Autodesk Inventor part; units mm, degrees
(part 2 of 4)
sketch "Sketch18" plane through (0, 4, 0) normal (0, 1, 0) x (1, 0, 0)
  line L0 (-39.75, -116.5) -> (-38.25, -116.5)
  line L1 (-38.25, -116.5) -> (-38.25, -108.5)
  line L2 (-38.25, -108.5) -> (-39.75, -108.5)
  line L3 (-39.75, -108.5) -> (-39.75, -116.5)
  line L4 (-41, -119.5) -> (-49.5, -119.5) projected
  line L5 (-41, -118) -> (-41, -119.5) projected
  line L6 (-24.75, -116.5) -> (-23.25, -116.5)
  line L7 (-23.25, -116.5) -> (-23.25, -108.5)
  line L8 (-23.25, -108.5) -> (-24.75, -108.5)
  line L9 (-24.75, -108.5) -> (-24.75, -116.5)
  line L10 (-9.75, -116.5) -> (-8.25, -116.5)
  line L11 (-8.25, -116.5) -> (-8.25, -108.5)
  line L12 (-8.25, -108.5) -> (-9.75, -108.5)
  line L13 (-9.75, -108.5) -> (-9.75, -116.5)
  line L14 (5.25, -116.5) -> (6.75, -116.5)
  line L15 (6.75, -116.5) -> (6.75, -108.5)
  line L16 (6.75, -108.5) -> (5.25, -108.5)
  line L17 (5.25, -108.5) -> (5.25, -116.5)
  line L18 (20.25, -116.5) -> (21.75, -116.5)
  line L19 (21.75, -116.5) -> (21.75, -108.5)
  line L20 (21.75, -108.5) -> (20.25, -108.5)
  line L21 (20.25, -108.5) -> (20.25, -116.5)
  line L22 (35.25, -116.5) -> (36.75, -116.5)
  line L23 (36.75, -116.5) -> (36.75, -108.5)
  line L24 (36.75, -108.5) -> (35.25, -108.5)
  line L25 (35.25, -108.5) -> (35.25, -116.5)
  line L26 (50.25, -116.5) -> (51.75, -116.5)
  line L27 (51.75, -116.5) -> (51.75, -108.5)
  line L28 (51.75, -108.5) -> (50.25, -108.5)
  line L29 (50.25, -108.5) -> (50.25, -116.5)
  line L30 (-39.75, -101.5) -> (-38.25, -101.5)
  line L31 (-38.25, -101.5) -> (-38.25, -93.5)
  line L32 (-38.25, -93.5) -> (-39.75, -93.5)
  line L33 (-39.75, -93.5) -> (-39.75, -101.5)
  line L34 (-24.75, -101.5) -> (-23.25, -101.5)
  line L35 (-23.25, -101.5) -> (-23.25, -93.5)
  line L36 (-23.25, -93.5) -> (-24.75, -93.5)
  line L37 (-24.75, -93.5) -> (-24.75, -101.5)
  line L38 (-9.75, -101.5) -> (-8.25, -101.5)
  line L39 (-8.25, -101.5) -> (-8.25, -93.5)
  line L40 (-8.25, -93.5) -> (-9.75, -93.5)
  line L41 (-9.75, -93.5) -> (-9.75, -101.5)
  line L42 (5.25, -101.5) -> (6.75, -101.5)
  line L43 (6.75, -101.5) -> (6.75, -93.5)
  line L44 (6.75, -93.5) -> (5.25, -93.5)
  line L45 (5.25, -93.5) -> (5.25, -101.5)
  line L46 (20.25, -101.5) -> (21.75, -101.5)
  line L47 (21.75, -101.5) -> (21.75, -93.5)
  line L48 (21.75, -93.5) -> (20.25, -93.5)
  line L49 (20.25, -93.5) -> (20.25, -101.5)
  line L50 (35.25, -101.5) -> (36.75, -101.5)
  line L51 (36.75, -101.5) -> (36.75, -93.5)
  line L52 (36.75, -93.5) -> (35.25, -93.5)
  line L53 (35.25, -93.5) -> (35.25, -101.5)
  line L54 (50.25, -101.5) -> (51.75, -101.5)
  line L55 (51.75, -101.5) -> (51.75, -93.5)
  line L56 (51.75, -93.5) -> (50.25, -93.5)
  line L57 (50.25, -93.5) -> (50.25, -101.5)
  line L58 (-39.75, -86.5) -> (-38.25, -86.5)
  line L59 (-38.25, -86.5) -> (-38.25, -78.5)
  line L60 (-38.25, -78.5) -> (-39.75, -78.5)
  line L61 (-39.75, -78.5) -> (-39.75, -86.5)
  line L62 (-24.75, -86.5) -> (-23.25, -86.5)
  line L63 (-23.25, -86.5) -> (-23.25, -78.5)
  line L64 (-23.25, -78.5) -> (-24.75, -78.5)
  line L65 (-24.75, -78.5) -> (-24.75, -86.5)
  line L66 (-9.75, -86.5) -> (-8.25, -86.5)
  line L67 (-8.25, -86.5) -> (-8.25, -78.5)
  line L68 (-8.25, -78.5) -> (-9.75, -78.5)
  line L69 (-9.75, -78.5) -> (-9.75, -86.5)
  line L70 (5.25, -86.5) -> (6.75, -86.5)
  line L71 (6.75, -86.5) -> (6.75, -78.5)
  line L72 (6.75, -78.5) -> (5.25, -78.5)
  line L73 (5.25, -78.5) -> (5.25, -86.5)
  line L74 (20.25, -86.5) -> (21.75, -86.5)
  line L75 (21.75, -86.5) -> (21.75, -78.5)
  line L76 (21.75, -78.5) -> (20.25, -78.5)
  line L77 (20.25, -78.5) -> (20.25, -86.5)
  line L78 (35.25, -86.5) -> (36.75, -86.5)
  line L79 (36.75, -86.5) -> (36.75, -78.5)
  line L80 (36.75, -78.5) -> (35.25, -78.5)
  line L81 (35.25, -78.5) -> (35.25, -86.5)
  line L82 (50.25, -86.5) -> (51.75, -86.5)
  line L83 (51.75, -86.5) -> (51.75, -78.5)
  line L84 (51.75, -78.5) -> (50.25, -78.5)
  line L85 (50.25, -78.5) -> (50.25, -86.5)
  line L86 (-39.75, -71.5) -> (-38.25, -71.5)
  line L87 (-38.25, -71.5) -> (-38.25, -63.5)
  line L88 (-38.25, -63.5) -> (-39.75, -63.5)
  line L89 (-39.75, -63.5) -> (-39.75, -71.5)
  line L90 (-24.75, -71.5) -> (-23.25, -71.5)
  line L91 (-23.25, -71.5) -> (-23.25, -63.5)
  line L92 (-23.25, -63.5) -> (-24.75, -63.5)
  line L93 (-24.75, -63.5) -> (-24.75, -71.5)
  line L94 (-9.75, -71.5) -> (-8.25, -71.5)
  line L95 (-8.25, -71.5) -> (-8.25, -63.5)
  line L96 (-8.25, -63.5) -> (-9.75, -63.5)
  line L97 (-9.75, -63.5) -> (-9.75, -71.5)
  line L98 (5.25, -71.5) -> (6.75, -71.5)
  line L99 (6.75, -71.5) -> (6.75, -63.5)
  line L100 (6.75, -63.5) -> (5.25, -63.5)
  line L101 (5.25, -63.5) -> (5.25, -71.5)
  line L102 (20.25, -71.5) -> (21.75, -71.5)
  line L103 (21.75, -71.5) -> (21.75, -63.5)
  line L104 (21.75, -63.5) -> (20.25, -63.5)
  line L105 (20.25, -63.5) -> (20.25, -71.5)
  line L106 (35.25, -71.5) -> (36.75, -71.5)
  line L107 (36.75, -71.5) -> (36.75, -63.5)
  line L108 (36.75, -63.5) -> (35.25, -63.5)
  line L109 (35.25, -63.5) -> (35.25, -71.5)
  line L110 (50.25, -71.5) -> (51.75, -71.5)
  line L111 (51.75, -71.5) -> (51.75, -63.5)
  line L112 (51.75, -63.5) -> (50.25, -63.5)
  line L113 (50.25, -63.5) -> (50.25, -71.5)
  line L114 (-39.75, -56.5) -> (-38.25, -56.5)
  line L115 (-38.25, -56.5) -> (-38.25, -48.5)
  line L116 (-38.25, -48.5) -> (-39.75, -48.5)
  line L117 (-39.75, -48.5) -> (-39.75, -56.5)
  line L118 (-24.75, -56.5) -> (-23.25, -56.5)
  line L119 (-23.25, -56.5) -> (-23.25, -48.5)
  line L120 (-23.25, -48.5) -> (-24.75, -48.5)
  line L121 (-24.75, -48.5) -> (-24.75, -56.5)
  line L122 (-9.75, -56.5) -> (-8.25, -56.5)
  line L123 (-8.25, -56.5) -> (-8.25, -48.5)
  line L124 (-8.25, -48.5) -> (-9.75, -48.5)
  line L125 (-9.75, -48.5) -> (-9.75, -56.5)
  line L126 (5.25, -56.5) -> (6.75, -56.5)
  line L127 (6.75, -56.5) -> (6.75, -48.5)
  line L128 (6.75, -48.5) -> (5.25, -48.5)
  line L129 (5.25, -48.5) -> (5.25, -56.5)
  line L130 (20.25, -56.5) -> (21.75, -56.5)
  line L131 (21.75, -56.5) -> (21.75, -48.5)
  line L132 (21.75, -48.5) -> (20.25, -48.5)
  line L133 (20.25, -48.5) -> (20.25, -56.5)
  line L134 (35.25, -56.5) -> (36.75, -56.5)
  line L135 (36.75, -56.5) -> (36.75, -48.5)
  line L136 (36.75, -48.5) -> (35.25, -48.5)
  line L137 (35.25, -48.5) -> (35.25, -56.5)
  line L138 (50.25, -56.5) -> (51.75, -56.5)
  line L139 (51.75, -56.5) -> (51.75, -48.5)
  line L140 (51.75, -48.5) -> (50.25, -48.5)
  line L141 (50.25, -48.5) -> (50.25, -56.5)
  line L142 (-39.75, -41.5) -> (-38.25, -41.5)
  line L143 (-38.25, -41.5) -> (-38.25, -33.5)
  line L144 (-38.25, -33.5) -> (-39.75, -33.5)
  line L145 (-39.75, -33.5) -> (-39.75, -41.5)
  line L146 (-24.75, -41.5) -> (-23.25, -41.5)
  line L147 (-23.25, -41.5) -> (-23.25, -33.5)
  line L148 (-23.25, -33.5) -> (-24.75, -33.5)
  line L149 (-24.75, -33.5) -> (-24.75, -41.5)
  line L150 (-9.75, -41.5) -> (-8.25, -41.5)
  line L151 (-8.25, -41.5) -> (-8.25, -33.5)
  line L152 (-8.25, -33.5) -> (-9.75, -33.5)
  line L153 (-9.75, -33.5) -> (-9.75, -41.5)
  line L154 (5.25, -41.5) -> (6.75, -41.5)
  line L155 (6.75, -41.5) -> (6.75, -33.5)
  line L156 (6.75, -33.5) -> (5.25, -33.5)
  line L157 (5.25, -33.5) -> (5.25, -41.5)
  line L158 (20.25, -41.5) -> (21.75, -41.5)
  line L159 (21.75, -41.5) -> (21.75, -33.5)
  line L160 (21.75, -33.5) -> (20.25, -33.5)
  line L161 (20.25, -33.5) -> (20.25, -41.5)
  line L162 (35.25, -41.5) -> (36.75, -41.5)
  line L163 (36.75, -41.5) -> (36.75, -33.5)
  line L164 (36.75, -33.5) -> (35.25, -33.5)
  line L165 (35.25, -33.5) -> (35.25, -41.5)
  line L166 (50.25, -41.5) -> (51.75, -41.5)
  line L167 (51.75, -41.5) -> (51.75, -33.5)
  line L168 (51.75, -33.5) -> (50.25, -33.5)
  line L169 (50.25, -33.5) -> (50.25, -41.5)
  line L170 (-39.75, -26.5) -> (-38.25, -26.5)
  line L171 (-38.25, -26.5) -> (-38.25, -18.5)
  line L172 (-38.25, -18.5) -> (-39.75, -18.5)
  line L173 (-39.75, -18.5) -> (-39.75, -26.5)
  line L174 (-24.75, -26.5) -> (-23.25, -26.5)
  line L175 (-23.25, -26.5) -> (-23.25, -18.5)
  line L176 (-23.25, -18.5) -> (-24.75, -18.5)
  line L177 (-24.75, -18.5) -> (-24.75, -26.5)
  line L178 (-9.75, -26.5) -> (-8.25, -26.5)
  line L179 (-8.25, -26.5) -> (-8.25, -18.5)
  line L180 (-8.25, -18.5) -> (-9.75, -18.5)
  line L181 (-9.75, -18.5) -> (-9.75, -26.5)
  line L182 (5.25, -26.5) -> (6.75, -26.5)
  line L183 (6.75, -26.5) -> (6.75, -18.5)
  line L184 (6.75, -18.5) -> (5.25, -18.5)
  line L185 (5.25, -18.5) -> (5.25, -26.5)
  line L186 (20.25, -26.5) -> (21.75, -26.5)
  line L187 (21.75, -26.5) -> (21.75, -18.5)
  line L188 (21.75, -18.5) -> (20.25, -18.5)
  line L189 (20.25, -18.5) -> (20.25, -26.5)
  line L190 (35.25, -26.5) -> (36.75, -26.5)
  line L191 (36.75, -26.5) -> (36.75, -18.5)
  line L192 (36.75, -18.5) -> (35.25, -18.5)
  line L193 (35.25, -18.5) -> (35.25, -26.5)
  line L194 (50.25, -26.5) -> (51.75, -26.5)
  line L195 (51.75, -26.5) -> (51.75, -18.5)
  line L196 (51.75, -18.5) -> (50.25, -18.5)
  line L197 (50.25, -18.5) -> (50.25, -26.5)
  line L198 (-39.75, -11.5) -> (-38.25, -11.5)
  line L199 (-38.25, -11.5) -> (-38.25, -3.5)
  line L200 (-38.25, -3.5) -> (-39.75, -3.5)
  line L201 (-39.75, -3.5) -> (-39.75, -11.5)
  line L202 (-24.75, -11.5) -> (-23.25, -11.5)
  line L203 (-23.25, -11.5) -> (-23.25, -3.5)
  line L204 (-23.25, -3.5) -> (-24.75, -3.5)
  line L205 (-24.75, -3.5) -> (-24.75, -11.5)
  line L206 (-9.75, -11.5) -> (-8.25, -11.5)
  line L207 (-8.25, -11.5) -> (-8.25, -3.5)
  line L208 (-8.25, -3.5) -> (-9.75, -3.5)
  line L209 (-9.75, -3.5) -> (-9.75, -11.5)
  line L210 (5.25, -11.5) -> (6.75, -11.5)
  line L211 (6.75, -11.5) -> (6.75, -3.5)
  line L212 (6.75, -3.5) -> (5.25, -3.5)
  line L213 (5.25, -3.5) -> (5.25, -11.5)
  line L214 (20.25, -11.5) -> (21.75, -11.5)
  line L215 (21.75, -11.5) -> (21.75, -3.5)
  line L216 (21.75, -3.5) -> (20.25, -3.5)
  line L217 (20.25, -3.5) -> (20.25, -11.5)
  line L218 (35.25, -11.5) -> (36.75, -11.5)
  line L219 (36.75, -11.5) -> (36.75, -3.5)
  line L220 (36.75, -3.5) -> (35.25, -3.5)
  line L221 (35.25, -3.5) -> (35.25, -11.5)
  line L222 (50.25, -11.5) -> (51.75, -11.5)
  line L223 (51.75, -11.5) -> (51.75, -3.5)
  line L224 (51.75, -3.5) -> (50.25, -3.5)
  line L225 (50.25, -3.5) -> (50.25, -11.5)
  line L226 (-39.75, 3.5) -> (-38.25, 3.5)
  line L227 (-38.25, 3.5) -> (-38.25, 11.5)
  line L228 (-38.25, 11.5) -> (-39.75, 11.5)
  line L229 (-39.75, 11.5) -> (-39.75, 3.5)
  line L230 (-24.75, 3.5) -> (-23.25, 3.5)
  line L231 (-23.25, 3.5) -> (-23.25, 11.5)
  line L232 (-23.25, 11.5) -> (-24.75, 11.5)
  line L233 (-24.75, 11.5) -> (-24.75, 3.5)
  line L234 (-9.75, 3.5) -> (-8.25, 3.5)
  line L235 (-8.25, 3.5) -> (-8.25, 11.5)
  line L236 (-8.25, 11.5) -> (-9.75, 11.5)
  line L237 (-9.75, 11.5) -> (-9.75, 3.5)
  line L238 (5.25, 3.5) -> (6.75, 3.5)
  line L239 (6.75, 3.5) -> (6.75, 11.5)
  line L240 (6.75, 11.5) -> (5.25, 11.5)
  line L241 (5.25, 11.5) -> (5.25, 3.5)
  line L242 (20.25, 3.5) -> (21.75, 3.5)
  line L243 (21.75, 3.5) -> (21.75, 11.5)
  line L244 (21.75, 11.5) -> (20.25, 11.5)
  line L245 (20.25, 11.5) -> (20.25, 3.5)
  line L246 (35.25, 3.5) -> (36.75, 3.5)
  line L247 (36.75, 3.5) -> (36.75, 11.5)
  line L248 (36.75, 11.5) -> (35.25, 11.5)
  line L249 (35.25, 11.5) -> (35.25, 3.5)
  line L250 (50.25, 3.5) -> (51.75, 3.5)
  line L251 (51.75, 3.5) -> (51.75, 11.5)
  line L252 (51.75, 11.5) -> (50.25, 11.5)
  line L253 (50.25, 11.5) -> (50.25, 3.5)
  line L254 (-39.75, 18.5) -> (-38.25, 18.5)
  line L255 (-38.25, 18.5) -> (-38.25, 26.5)
  line L256 (-38.25, 26.5) -> (-39.75, 26.5)
  line L257 (-39.75, 26.5) -> (-39.75, 18.5)
  line L258 (-24.75, 18.5) -> (-23.25, 18.5)
  line L259 (-23.25, 18.5) -> (-23.25, 26.5)
  line L260 (-23.25, 26.5) -> (-24.75, 26.5)
  line L261 (-24.75, 26.5) -> (-24.75, 18.5)
  line L262 (-9.75, 18.5) -> (-8.25, 18.5)
  line L263 (-8.25, 18.5) -> (-8.25, 26.5)
  line L264 (-8.25, 26.5) -> (-9.75, 26.5)
  line L265 (-9.75, 26.5) -> (-9.75, 18.5)
  line L266 (5.25, 18.5) -> (6.75, 18.5)
  line L267 (6.75, 18.5) -> (6.75, 26.5)
  line L268 (6.75, 26.5) -> (5.25, 26.5)
  line L269 (5.25, 26.5) -> (5.25, 18.5)
  line L270 (20.25, 18.5) -> (21.75, 18.5)
  line L271 (21.75, 18.5) -> (21.75, 26.5)
  line L272 (21.75, 26.5) -> (20.25, 26.5)
  line L273 (20.25, 26.5) -> (20.25, 18.5)
  line L274 (35.25, 18.5) -> (36.75, 18.5)
  line L275 (36.75, 18.5) -> (36.75, 26.5)
  line L276 (36.75, 26.5) -> (35.25, 26.5)
  line L277 (35.25, 26.5) -> (35.25, 18.5)
  line L278 (50.25, 18.5) -> (51.75, 18.5)
  line L279 (51.75, 18.5) -> (51.75, 26.5)
  line L280 (51.75, 26.5) -> (50.25, 26.5)
  line L281 (50.25, 26.5) -> (50.25, 18.5)
  line L282 (-39.75, 33.5) -> (-38.25, 33.5)
  line L283 (-38.25, 33.5) -> (-38.25, 41.5)
  line L284 (-38.25, 41.5) -> (-39.75, 41.5)
  line L285 (-39.75, 41.5) -> (-39.75, 33.5)
  line L286 (-24.75, 33.5) -> (-23.25, 33.5)
  line L287 (-23.25, 33.5) -> (-23.25, 41.5)
  line L288 (-23.25, 41.5) -> (-24.75, 41.5)
  line L289 (-24.75, 41.5) -> (-24.75, 33.5)
  line L290 (-9.75, 33.5) -> (-8.25, 33.5)
  line L291 (-8.25, 33.5) -> (-8.25, 41.5)
  line L292 (-8.25, 41.5) -> (-9.75, 41.5)
  line L293 (-9.75, 41.5) -> (-9.75, 33.5)
  line L294 (5.25, 33.5) -> (6.75, 33.5)
  line L295 (6.75, 33.5) -> (6.75, 41.5)
  line L296 (6.75, 41.5) -> (5.25, 41.5)
  line L297 (5.25, 41.5) -> (5.25, 33.5)
  line L298 (20.25, 33.5) -> (21.75, 33.5)
  line L299 (21.75, 33.5) -> (21.75, 41.5)
  line L300 (21.75, 41.5) -> (20.25, 41.5)
  line L301 (20.25, 41.5) -> (20.25, 33.5)
  line L302 (35.25, 33.5) -> (36.75, 33.5)
  line L303 (36.75, 33.5) -> (36.75, 41.5)
  line L304 (36.75, 41.5) -> (35.25, 41.5)
  line L305 (35.25, 41.5) -> (35.25, 33.5)
  line L306 (50.25, 33.5) -> (51.75, 33.5)
  line L307 (51.75, 33.5) -> (51.75, 41.5)
  line L308 (51.75, 41.5) -> (50.25, 41.5)
  line L309 (50.25, 41.5) -> (50.25, 33.5)
  line L310 (-39.75, 48.5) -> (-38.25, 48.5)
  line L311 (-38.25, 48.5) -> (-38.25, 56.5)
  line L312 (-38.25, 56.5) -> (-39.75, 56.5)
  line L313 (-39.75, 56.5) -> (-39.75, 48.5)
  line L314 (-24.75, 48.5) -> (-23.25, 48.5)
  line L315 (-23.25, 48.5) -> (-23.25, 56.5)
  line L316 (-23.25, 56.5) -> (-24.75, 56.5)
  line L317 (-24.75, 56.5) -> (-24.75, 48.5)
  line L318 (-9.75, 48.5) -> (-8.25, 48.5)
  line L319 (-8.25, 48.5) -> (-8.25, 56.5)
  line L320 (-8.25, 56.5) -> (-9.75, 56.5)
  line L321 (-9.75, 56.5) -> (-9.75, 48.5)
  line L322 (5.25, 48.5) -> (6.75, 48.5)
  line L323 (6.75, 48.5) -> (6.75, 56.5)
  line L324 (6.75, 56.5) -> (5.25, 56.5)
  line L325 (5.25, 56.5) -> (5.25, 48.5)
  line L326 (20.25, 48.5) -> (21.75, 48.5)
  line L327 (21.75, 48.5) -> (21.75, 56.5)
  line L328 (21.75, 56.5) -> (20.25, 56.5)
  line L329 (20.25, 56.5) -> (20.25, 48.5)
  line L330 (35.25, 48.5) -> (36.75, 48.5)
  line L331 (36.75, 48.5) -> (36.75, 56.5)
  line L332 (36.75, 56.5) -> (35.25, 56.5)
  line L333 (35.25, 56.5) -> (35.25, 48.5)
  line L334 (50.25, 48.5) -> (51.75, 48.5)
  line L335 (51.75, 48.5) -> (51.75, 56.5)
  line L336 (51.75, 56.5) -> (50.25, 56.5)
  line L337 (50.25, 56.5) -> (50.25, 48.5)
  line L338 (-39.75, 63.5) -> (-38.25, 63.5)
  line L339 (-38.25, 63.5) -> (-38.25, 71.5)
  line L340 (-38.25, 71.5) -> (-39.75, 71.5)
  line L341 (-39.75, 71.5) -> (-39.75, 63.5)
  line L342 (-24.75, 63.5) -> (-23.25, 63.5)
  line L343 (-23.25, 63.5) -> (-23.25, 71.5)
  line L344 (-23.25, 71.5) -> (-24.75, 71.5)
  line L345 (-24.75, 71.5) -> (-24.75, 63.5)
  line L346 (-9.75, 63.5) -> (-8.25, 63.5)
  line L347 (-8.25, 63.5) -> (-8.25, 71.5)
  line L348 (-8.25, 71.5) -> (-9.75, 71.5)
  line L349 (-9.75, 71.5) -> (-9.75, 63.5)
  line L350 (5.25, 63.5) -> (6.75, 63.5)
  line L351 (6.75, 63.5) -> (6.75, 71.5)
  line L352 (6.75, 71.5) -> (5.25, 71.5)
  line L353 (5.25, 71.5) -> (5.25, 63.5)
  line L354 (20.25, 63.5) -> (21.75, 63.5)
  line L355 (21.75, 63.5) -> (21.75, 71.5)
  line L356 (21.75, 71.5) -> (20.25, 71.5)
  line L357 (20.25, 71.5) -> (20.25, 63.5)
  line L358 (35.25, 63.5) -> (36.75, 63.5)
  line L359 (36.75, 63.5) -> (36.75, 71.5)
  line L360 (36.75, 71.5) -> (35.25, 71.5)
  line L361 (35.25, 71.5) -> (35.25, 63.5)
  line L362 (50.25, 63.5) -> (51.75, 63.5)
  line L363 (51.75, 63.5) -> (51.75, 71.5)
  line L364 (51.75, 71.5) -> (50.25, 71.5)
  line L365 (50.25, 71.5) -> (50.25, 63.5)
  line L366 (-39.75, 78.5) -> (-38.25, 78.5)
  line L367 (-38.25, 78.5) -> (-38.25, 86.5)
  line L368 (-38.25, 86.5) -> (-39.75, 86.5)
  line L369 (-39.75, 86.5) -> (-39.75, 78.5)
  line L370 (-24.75, 78.5) -> (-23.25, 78.5)
  line L371 (-23.25, 78.5) -> (-23.25, 86.5)
  line L372 (-23.25, 86.5) -> (-24.75, 86.5)
  line L373 (-24.75, 86.5) -> (-24.75, 78.5)
  line L374 (-9.75, 78.5) -> (-8.25, 78.5)
  line L375 (-8.25, 78.5) -> (-8.25, 86.5)
  line L376 (-8.25, 86.5) -> (-9.75, 86.5)
  line L377 (-9.75, 86.5) -> (-9.75, 78.5)
  line L378 (5.25, 78.5) -> (6.75, 78.5)
  line L379 (6.75, 78.5) -> (6.75, 86.5)
  line L380 (6.75, 86.5) -> (5.25, 86.5)
  line L381 (5.25, 86.5) -> (5.25, 78.5)
  line L382 (20.25, 78.5) -> (21.75, 78.5)
  line L383 (21.75, 78.5) -> (21.75, 86.5)
  line L384 (21.75, 86.5) -> (20.25, 86.5)
  line L385 (20.25, 86.5) -> (20.25, 78.5)
  line L386 (35.25, 78.5) -> (36.75, 78.5)
  line L387 (36.75, 78.5) -> (36.75, 86.5)
  line L388 (36.75, 86.5) -> (35.25, 86.5)
  line L389 (35.25, 86.5) -> (35.25, 78.5)
  line L390 (50.25, 78.5) -> (51.75, 78.5)
  line L391 (51.75, 78.5) -> (51.75, 86.5)
  line L392 (51.75, 86.5) -> (50.25, 86.5)
  line L393 (50.25, 86.5) -> (50.25, 78.5)
  line L394 (-39.75, 93.5) -> (-38.25, 93.5)
  line L395 (-38.25, 93.5) -> (-38.25, 101.5)
  line L396 (-38.25, 101.5) -> (-39.75, 101.5)
  line L397 (-39.75, 101.5) -> (-39.75, 93.5)
  line L398 (-24.75, 93.5) -> (-23.25, 93.5)
  line L399 (-23.25, 93.5) -> (-23.25, 101.5)
  line L400 (-23.25, 101.5) -> (-24.75, 101.5)
  line L401 (-24.75, 101.5) -> (-24.75, 93.5)
  line L402 (-9.75, 93.5) -> (-8.25, 93.5)
  line L403 (-8.25, 93.5) -> (-8.25, 101.5)
  line L404 (-8.25, 101.5) -> (-9.75, 101.5)
  line L405 (-9.75, 101.5) -> (-9.75, 93.5)
  line L406 (5.25, 93.5) -> (6.75, 93.5)
  line L407 (6.75, 93.5) -> (6.75, 101.5)
  line L408 (6.75, 101.5) -> (5.25, 101.5)
  line L409 (5.25, 101.5) -> (5.25, 93.5)
  line L410 (20.25, 93.5) -> (21.75, 93.5)
  line L411 (21.75, 93.5) -> (21.75, 101.5)
  line L412 (21.75, 101.5) -> (20.25, 101.5)
  line L413 (20.25, 101.5) -> (20.25, 93.5)
  line L414 (35.25, 93.5) -> (36.75, 93.5)
  line L415 (36.75, 93.5) -> (36.75, 101.5)
  line L416 (36.75, 101.5) -> (35.25, 101.5)
  line L417 (35.25, 101.5) -> (35.25, 93.5)
  line L418 (50.25, 93.5) -> (51.75, 93.5)
  line L419 (51.75, 93.5) -> (51.75, 101.5)
  line L420 (51.75, 101.5) -> (50.25, 101.5)
  line L421 (50.25, 101.5) -> (50.25, 93.5)
  line L422 (-39.75, 108.5) -> (-38.25, 108.5)
  line L423 (-38.25, 108.5) -> (-38.25, 116.5)
  line L424 (-38.25, 116.5) -> (-39.75, 116.5)
  line L425 (-39.75, 116.5) -> (-39.75, 108.5)
  line L426 (-24.75, 108.5) -> (-23.25, 108.5)
  line L427 (-23.25, 108.5) -> (-23.25, 116.5)
  line L428 (-23.25, 116.5) -> (-24.75, 116.5)
  line L429 (-24.75, 116.5) -> (-24.75, 108.5)
  line L430 (-9.75, 108.5) -> (-8.25, 108.5)
  line L431 (-8.25, 108.5) -> (-8.25, 116.5)
  line L432 (-8.25, 116.5) -> (-9.75, 116.5)
  line L433 (-9.75, 116.5) -> (-9.75, 108.5)
  line L434 (5.25, 108.5) -> (6.75, 108.5)
  line L435 (6.75, 108.5) -> (6.75, 116.5)
  line L436 (6.75, 116.5) -> (5.25, 116.5)
  line L437 (5.25, 116.5) -> (5.25, 108.5)
  line L438 (20.25, 108.5) -> (21.75, 108.5)
  line L439 (21.75, 108.5) -> (21.75, 116.5)
  line L440 (21.75, 116.5) -> (20.25, 116.5)
  line L441 (20.25, 116.5) -> (20.25, 108.5)
  line L442 (35.25, 108.5) -> (36.75, 108.5)
  line L443 (36.75, 108.5) -> (36.75, 116.5)
  line L444 (36.75, 116.5) -> (35.25, 116.5)
  line L445 (35.25, 116.5) -> (35.25, 108.5)
  line L446 (50.25, 108.5) -> (51.75, 108.5)
  line L447 (51.75, 108.5) -> (51.75, 116.5)
  line L448 (51.75, 116.5) -> (50.25, 116.5)
  line L449 (50.25, 116.5) -> (50.25, 108.5)
  line L450 (19, -89.5) -> (10.5, -89.5) projected
  line L451 (20.25, -82.75) -> (21.75, -82.75)
  line L452 (21.75, -82.75) -> (21.75, -74.75)
  line L453 (21.75, -74.75) -> (20.25, -74.75)
  line L454 (20.25, -74.75) -> (20.25, -82.75)
  line L455 (20.25, -60.25) -> (21.75, -60.25)
  line L456 (21.75, -60.25) -> (21.75, -52.25)
  line L457 (21.75, -52.25) -> (20.25, -52.25)
  line L458 (20.25, -52.25) -> (20.25, -60.25)
  line L459 (20.25, -37.75) -> (21.75, -37.75)
  line L460 (21.75, -37.75) -> (21.75, -29.75)
  line L461 (21.75, -29.75) -> (20.25, -29.75)
  line L462 (20.25, -29.75) -> (20.25, -37.75)
  line L463 (19, -44.5) -> (10.5, -44.5) projected
  line L464 (20.25, -19) -> (21.75, -19)
  line L465 (21.75, -19) -> (21.75, -11)
  line L466 (21.75, -11) -> (20.25, -11)
  line L467 (20.25, -11) -> (20.25, -19)
  line L468 (10.5, -20.5) -> (19, -20.5) projected
  line L469 (19, -22) -> (10.5, -22) projected
  line L470 (19, -8) -> (19, -9.5) projected
  line L471 (20.25, -0.25) -> (21.75, -0.25)
  line L472 (21.75, -0.25) -> (21.75, 7.75)
  line L473 (21.75, 7.75) -> (20.25, 7.75)
  line L474 (20.25, 7.75) -> (20.25, -0.25)
  line L475 (20.25, 22.25) -> (21.75, 22.25)
  line L476 (21.75, 22.25) -> (21.75, 30.25)
  line L477 (21.75, 30.25) -> (20.25, 30.25)
  line L478 (20.25, 30.25) -> (20.25, 22.25)
  line L479 (20.25, 44.75) -> (21.75, 44.75)
  line L480 (21.75, 44.75) -> (21.75, 52.75)
  line L481 (21.75, 52.75) -> (20.25, 52.75)
  line L482 (20.25, 52.75) -> (20.25, 44.75)
  line L483 (20.25, 67.25) -> (21.75, 67.25)
  line L484 (21.75, 67.25) -> (21.75, 75.25)
  line L485 (21.75, 75.25) -> (20.25, 75.25)
  line L486 (20.25, 75.25) -> (20.25, 67.25)
  line L487 (20.25, 86) -> (21.75, 86)
  line L488 (21.75, 86) -> (21.75, 94)
  line L489 (21.75, 94) -> (20.25, 94)
  line L490 (20.25, 94) -> (20.25, 86)
  line L491 (20.25, 104.75) -> (21.75, 104.75)
  line L492 (21.75, 104.75) -> (21.75, 112.75)
  line L493 (21.75, 112.75) -> (20.25, 112.75)
  line L494 (20.25, 112.75) -> (20.25, 104.75)
  line L495 (19, 83) -> (10.5, 83) projected
  line L496 (19, 60.5) -> (10.5, 60.5) projected
  line L497 (10.5, 59.5) -> (19, 59.5) projected
  line L498 (10.5, 14.5) -> (19, 14.5) projected
  line L499 (10.5, -45.5) -> (19, -45.5) projected
  line L500 (19, 98) -> (10.5, 98) projected
  line L501 (10.5, 37) -> (19, 37) projected
  point P0 (0, 0)
  point P1 (20.25, -81.75)
  point P2 (20.25, -63)
  point P3 (21.75, -55)
  point P4 (20.25, -36.25)
  point P5 (20.25, -21.75)
  point P6 (20.25, -7)
  point P7 (20.25, 8.75)
  point P8 (21.75, 0.75)
  point P9 (20.25, 23.25)
  point P10 (21.75, 31.25)
  point P11 (20.25, 42)
  point P12 (21.75, 50)
  point P13 (20.25, 68.75)
  point P14 (21.75, 60.75)
  point P15 (20.25, 83.25)
  point P16 (21.75, 113.75)
  point P17 (20.25, 112.75)
  point P18 (20.25, 108.5)
  point P19 (21.75, 108.5)
  point P20 (20.25, 86)
  point P21 (21.75, 86)
  point P22 (21.75, 86.5)
  point P23 (21.75, 93.5)
  point P24 (21.75, 94)
  point P25 (20.25, 94)
  point P26 (20.25, 93.5)
  point P27 (20.25, 86.5)
  point P28 (21.75, 67.25)
  point P29 (21.75, 71.5)
  point P30 (20.25, 71.5)
  point P31 (20.25, 52.75)
  point P32 (20.25, 48.5)
  point P33 (21.75, 48.5)
  point P34 (21.75, 22.25)
  point P35 (21.75, 26.5)
  point P36 (20.25, 26.5)
  point P37 (20.25, 7.75)
  point P38 (20.25, 3.5)
  point P39 (21.75, 3.5)
  point P40 (20.25, -19)
  point P41 (21.75, -19)
  point P42 (21.75, -18.5)
  point P43 (21.75, -11.5)
  point P44 (21.75, -11)
  point P45 (20.25, -11)
  point P46 (20.25, -11.5)
  point P47 (20.25, -18.5)
  point P48 (21.75, -37.75)
  point P49 (21.75, -33.5)
  point P50 (20.25, -33.5)
  point P51 (20.25, -52.25)
  point P52 (20.25, -56.5)
  point P53 (21.75, -56.5)
  point P54 (21.75, -82.75)
  point P55 (21.75, -78.5)
  point P56 (20.25, -78.5)
  dimension "d177" = 8
  dimension "d178" = 1.5
  dimension "d179" = 3
  dimension "d180" = 1.25
  dimension "d187" = 15
  dimension "d190" = 15
  dimension "d296" = 6.75
  dimension "d297" = 8
  dimension "d298" = 1.5
  dimension "d300" = 8
  dimension "d301" = 6.75
  dimension "d302" = 8
  dimension "d303" = 1.5
  dimension "d304" = 8
  dimension "d306" = 3
  dimension "d307" = 1.5
  dimension "d308" = 1.25
  dimension "d309" = 8
  dimension "d310" = 8
  dimension "d311" = 8
  dimension "d312" = 8
  dimension "d313" = 8
  dimension "d314" = 8
  dimension "d316" = 3
  dimension "d317" = 6.75
  dimension "d318" = 6.75
  dimension "d320" = 6.75
  dimension "d321" = 1.5
  dimension "d323" = 6.75
  dimension "d324" = 6.75
  dimension "d325" = 6.75
  constraints: 976 end point, 30 point on line, 22 parallel, 12 horizontal, 11 perpendicular, 1 vertical, 889 other
  measures "d177" distance of L2.end L0.start
  measures "d178" distance of L1.end L2.end
  measures "d179" distance between parallel lines of L4 L0
  measures "d180" distance between parallel lines of L5 L3
  measures "d187" distance of L0.start L6.start
  measures "d190" distance of L0.start L30.start
  measures "d296" distance between parallel lines of L450 L451
  measures "d297" distance of L451.end L452.end
  measures "d298" distance of L452.end L453.end
  measures "d300" distance of L455.end L456.end
  measures "d301" distance between parallel lines of L463 L459
  measures "d302" distance of L459.end L460.end
  measures "d303" distance of L460.end L461.end
  measures "d304" distance of L464.end L465.end
  measures "d306" distance between parallel lines of L469 L464
  measures "d307" distance of L465.end L466.end
  measures "d309" distance of L471.end L472.end
  measures "d310" distance of L475.end L476.end
  measures "d311" distance of L479.end L480.end
  measures "d312" distance of L483.end L484.end
  measures "d313" distance of L487.end L488.end
  measures "d314" distance of L491.end L492.end
  measures "d316" distance between parallel lines of L495 L487
  measures "d317" distance between parallel lines of L496 L483
  measures "d318" distance between parallel lines of L497 L481
  measures "d320" distance between parallel lines of L498 L473
  measures "d321" distance of L471.start L471.end
  measures "d323" distance between parallel lines of L499 L457
  measures "d324" distance between parallel lines of L500 L491
  measures "d325" distance between parallel lines of L501 L477
extrude "Extrusion7" cut sketch "Sketch18" against normal blind 8 contours L3 L2 L1 L0 | L9 L8 L7 L6 | L13 L12 L11 L10 | L17 L16 L15 L14 | L21 L20 L19 L18 | L25 L24 L23 L22 | L29 L28 L27 L26 | L33 L32 L31 L30 | L37 L36 L35 L34 | L41 L40 L39 L38 | L45 L44 L43 L42 | L49 L48 L47 L46 | L53 L52 L51 L50 | L57 L56 L55 L54 | L77 L76 L75 L451 | L454 L453 L452 L76 | L85 L84 L83 L82 | L113 L112 L111 L110 | L133 L457 L131 L130 | L130 L456 L455 L458 | L141 L140 L139 L138 | L161 L160 L159 L459 | L462 L461 L460 L160 | L169 L168 L167 L166 | L189 L188 L187 L464 | L467 L214 L465 L188 | L217 L466 L215 L214 | L197 L196 L195 L194 | L225 L224 L223 L222 | L237 L236 L235 L234 | L241 L240 L239 L238 | L245 L473 L243 L242 | L242 L472 L471 L474 | L253 L252 L251 L250 | L265 L264 L263 L262 | L269 L268 L267 L266 | L273 L272 L271 L475 | L478 L477 L476 L272 | L281 L280 L279 L278 | L293 L292 L291 L290 | L297 L296 L295 L294 | L309 L308 L307 L306 | L321 L320 L319 L318 | L325 L324 L323 L322 | L329 L481 L327 L326 | L326 L480 L479 L482 | L337 L336 L335 L334 | L349 L348 L347 L346 | L353 L352 L351 L350 | L357 L356 L355 L483 | L486 L485 L484 L356 | L365 L364 L363 L362 | L377 L376 L375 L374 | L381 L380 L379 L378 | L385 L384 L383 L487 | L490 L410 L488 L384 | L413 L489 L411 L410 | L393 L392 L391 L390 | L405 L404 L403 L402 | L409 L408 L407 L406 | L421 L420 L419 L418 | L433 L432 L431 L430 | L437 L436 L435 L434 | L441 L493 L439 L438 | L438 L492 L491 L494 | L449 L448 L447 L446
sketch "Sketch21" plane through (0, 4, 0) normal (0, 1, 0) x (1, 0, 0)
  line L0 (-40, -117.75) -> (-50.5, -117.75)
  line L1 (-50.5, -117.75) -> (-50.5, -107.25)
  line L2 (-50.5, -107.25) -> (-40, -107.25)
  line L3 (-40, -107.25) -> (-40, -117.75)
  line L4 (-49.5, -118) -> (-41, -118) projected
  line L5 (-39.75, -116.5) -> (-39.75, -108.5) projected
  line L6 (-40, -102.75) -> (-50.5, -102.75)
  line L7 (-50.5, -102.75) -> (-50.5, -92.25)
  line L8 (-50.5, -92.25) -> (-40, -92.25)
  line L9 (-40, -92.25) -> (-40, -102.75)
  line L10 (-40, -87.75) -> (-50.5, -87.75)
  line L11 (-50.5, -87.75) -> (-50.5, -77.25)
  line L12 (-50.5, -77.25) -> (-40, -77.25)
  line L13 (-40, -77.25) -> (-40, -87.75)
  line L14 (-40, -72.75) -> (-50.5, -72.75)
  line L15 (-50.5, -72.75) -> (-50.5, -62.25)
  line L16 (-50.5, -62.25) -> (-40, -62.25)
  line L17 (-40, -62.25) -> (-40, -72.75)
  line L18 (-40, -57.75) -> (-50.5, -57.75)
  line L19 (-50.5, -57.75) -> (-50.5, -47.25)
  line L20 (-50.5, -47.25) -> (-40, -47.25)
  line L21 (-40, -47.25) -> (-40, -57.75)
  line L22 (-40, -42.75) -> (-50.5, -42.75)
  line L23 (-50.5, -42.75) -> (-50.5, -32.25)
  line L24 (-50.5, -32.25) -> (-40, -32.25)
  line L25 (-40, -32.25) -> (-40, -42.75)
  line L26 (-40, -27.75) -> (-50.5, -27.75)
  line L27 (-50.5, -27.75) -> (-50.5, -17.25)
  line L28 (-50.5, -17.25) -> (-40, -17.25)
  line L29 (-40, -17.25) -> (-40, -27.75)
  line L30 (-40, -12.75) -> (-50.5, -12.75)
  line L31 (-50.5, -12.75) -> (-50.5, -2.25)
  line L32 (-50.5, -2.25) -> (-40, -2.25)
  line L33 (-40, -2.25) -> (-40, -12.75)
  line L34 (-40, 2.25) -> (-50.5, 2.25)
  line L35 (-50.5, 2.25) -> (-50.5, 12.75)
  line L36 (-50.5, 12.75) -> (-40, 12.75)
  line L37 (-40, 12.75) -> (-40, 2.25)
  line L38 (-40, 17.25) -> (-50.5, 17.25)
  line L39 (-50.5, 17.25) -> (-50.5, 27.75)
  line L40 (-50.5, 27.75) -> (-40, 27.75)
  line L41 (-40, 27.75) -> (-40, 17.25)
  line L42 (-40, 32.25) -> (-50.5, 32.25)
  line L43 (-50.5, 32.25) -> (-50.5, 42.75)
  line L44 (-50.5, 42.75) -> (-40, 42.75)
  line L45 (-40, 42.75) -> (-40, 32.25)
  line L46 (-40, 47.25) -> (-50.5, 47.25)
  line L47 (-50.5, 47.25) -> (-50.5, 57.75)
  line L48 (-50.5, 57.75) -> (-40, 57.75)
  line L49 (-40, 57.75) -> (-40, 47.25)
  line L50 (-40, 62.25) -> (-50.5, 62.25)
  line L51 (-50.5, 62.25) -> (-50.5, 72.75)
  line L52 (-50.5, 72.75) -> (-40, 72.75)
  line L53 (-40, 72.75) -> (-40, 62.25)
  line L54 (-40, 77.25) -> (-50.5, 77.25)
  line L55 (-50.5, 77.25) -> (-50.5, 87.75)
  line L56 (-50.5, 87.75) -> (-40, 87.75)
  line L57 (-40, 87.75) -> (-40, 77.25)
  line L58 (-40, 92.25) -> (-50.5, 92.25)
  line L59 (-50.5, 92.25) -> (-50.5, 102.75)
  line L60 (-50.5, 102.75) -> (-40, 102.75)
  line L61 (-40, 102.75) -> (-40, 92.25)
  line L62 (-40, 107.25) -> (-50.5, 107.25)
  line L63 (-50.5, 107.25) -> (-50.5, 117.75)
  line L64 (-50.5, 117.75) -> (-40, 117.75)
  line L65 (-40, 117.75) -> (-40, 107.25)
  line L66 (-25, -117.75) -> (-35.5, -117.75)
  line L67 (-35.5, -117.75) -> (-35.5, -107.25)
  line L68 (-35.5, -107.25) -> (-25, -107.25)
  line L69 (-25, -107.25) -> (-25, -117.75)
  line L70 (-25, -102.75) -> (-35.5, -102.75)
  line L71 (-35.5, -102.75) -> (-35.5, -92.25)
  line L72 (-35.5, -92.25) -> (-25, -92.25)
  line L73 (-25, -92.25) -> (-25, -102.75)
  line L74 (-25, -87.75) -> (-35.5, -87.75)
  line L75 (-35.5, -87.75) -> (-35.5, -77.25)
  line L76 (-35.5, -77.25) -> (-25, -77.25)
  line L77 (-25, -77.25) -> (-25, -87.75)
  line L78 (-25, -72.75) -> (-35.5, -72.75)
  line L79 (-35.5, -72.75) -> (-35.5, -62.25)
  line L80 (-35.5, -62.25) -> (-25, -62.25)
  line L81 (-25, -62.25) -> (-25, -72.75)
  line L82 (-25, -57.75) -> (-35.5, -57.75)
  line L83 (-35.5, -57.75) -> (-35.5, -47.25)
  line L84 (-35.5, -47.25) -> (-25, -47.25)
  line L85 (-25, -47.25) -> (-25, -57.75)
  line L86 (-25, -42.75) -> (-35.5, -42.75)
  line L87 (-35.5, -42.75) -> (-35.5, -32.25)
  line L88 (-35.5, -32.25) -> (-25, -32.25)
  line L89 (-25, -32.25) -> (-25, -42.75)
  line L90 (-25, -27.75) -> (-35.5, -27.75)
  line L91 (-35.5, -27.75) -> (-35.5, -17.25)
  line L92 (-35.5, -17.25) -> (-25, -17.25)
  line L93 (-25, -17.25) -> (-25, -27.75)
  line L94 (-25, -12.75) -> (-35.5, -12.75)
  line L95 (-35.5, -12.75) -> (-35.5, -2.25)
  line L96 (-35.5, -2.25) -> (-25, -2.25)
  line L97 (-25, -2.25) -> (-25, -12.75)
  line L98 (-25, 2.25) -> (-35.5, 2.25)
  line L99 (-35.5, 2.25) -> (-35.5, 12.75)
  line L100 (-35.5, 12.75) -> (-25, 12.75)
  line L101 (-25, 12.75) -> (-25, 2.25)
  line L102 (-25, 17.25) -> (-35.5, 17.25)
  line L103 (-35.5, 17.25) -> (-35.5, 27.75)
  line L104 (-35.5, 27.75) -> (-25, 27.75)
  line L105 (-25, 27.75) -> (-25, 17.25)
  line L106 (-25, 32.25) -> (-35.5, 32.25)
  line L107 (-35.5, 32.25) -> (-35.5, 42.75)
  line L108 (-35.5, 42.75) -> (-25, 42.75)
  line L109 (-25, 42.75) -> (-25, 32.25)
  line L110 (-25, 47.25) -> (-35.5, 47.25)
  line L111 (-35.5, 47.25) -> (-35.5, 57.75)
  line L112 (-35.5, 57.75) -> (-25, 57.75)
  line L113 (-25, 57.75) -> (-25, 47.25)
  line L114 (-25, 62.25) -> (-35.5, 62.25)
  line L115 (-35.5, 62.25) -> (-35.5, 72.75)
  line L116 (-35.5, 72.75) -> (-25, 72.75)
  line L117 (-25, 72.75) -> (-25, 62.25)
  line L118 (-25, 77.25) -> (-35.5, 77.25)
  line L119 (-35.5, 77.25) -> (-35.5, 87.75)
  line L120 (-35.5, 87.75) -> (-25, 87.75)
  line L121 (-25, 87.75) -> (-25, 77.25)
  line L122 (-25, 92.25) -> (-35.5, 92.25)
  line L123 (-35.5, 92.25) -> (-35.5, 102.75)
  line L124 (-35.5, 102.75) -> (-25, 102.75)
  line L125 (-25, 102.75) -> (-25, 92.25)
  line L126 (-25, 107.25) -> (-35.5, 107.25)
  line L127 (-35.5, 107.25) -> (-35.5, 117.75)
  line L128 (-35.5, 117.75) -> (-25, 117.75)
  line L129 (-25, 117.75) -> (-25, 107.25)
  line L130 (-10, -117.75) -> (-20.5, -117.75)
  line L131 (-20.5, -117.75) -> (-20.5, -107.25)
  line L132 (-20.5, -107.25) -> (-10, -107.25)
  line L133 (-10, -107.25) -> (-10, -117.75)
  line L134 (-10, -102.75) -> (-20.5, -102.75)
  line L135 (-20.5, -102.75) -> (-20.5, -92.25)
  line L136 (-20.5, -92.25) -> (-10, -92.25)
  line L137 (-10, -92.25) -> (-10, -102.75)
  line L138 (-10, -87.75) -> (-20.5, -87.75)
  line L139 (-20.5, -87.75) -> (-20.5, -77.25)
  line L140 (-20.5, -77.25) -> (-10, -77.25)
  line L141 (-10, -77.25) -> (-10, -87.75)
  line L142 (-10, -72.75) -> (-20.5, -72.75)
  line L143 (-20.5, -72.75) -> (-20.5, -62.25)
  line L144 (-20.5, -62.25) -> (-10, -62.25)
  line L145 (-10, -62.25) -> (-10, -72.75)
  line L146 (-10, -57.75) -> (-20.5, -57.75)
  line L147 (-20.5, -57.75) -> (-20.5, -47.25)
  line L148 (-20.5, -47.25) -> (-10, -47.25)
  line L149 (-10, -47.25) -> (-10, -57.75)
  line L150 (-10, -42.75) -> (-20.5, -42.75)
  line L151 (-20.5, -42.75) -> (-20.5, -32.25)
  line L152 (-20.5, -32.25) -> (-10, -32.25)
  line L153 (-10, -32.25) -> (-10, -42.75)
  line L154 (-10, -27.75) -> (-20.5, -27.75)
  line L155 (-20.5, -27.75) -> (-20.5, -17.25)
  line L156 (-20.5, -17.25) -> (-10, -17.25)
  line L157 (-10, -17.25) -> (-10, -27.75)
  line L158 (-10, -12.75) -> (-20.5, -12.75)
  line L159 (-20.5, -12.75) -> (-20.5, -2.25)
  line L160 (-20.5, -2.25) -> (-10, -2.25)
  line L161 (-10, -2.25) -> (-10, -12.75)
  line L162 (-10, 2.25) -> (-20.5, 2.25)
  line L163 (-20.5, 2.25) -> (-20.5, 12.75)
  line L164 (-20.5, 12.75) -> (-10, 12.75)
  line L165 (-10, 12.75) -> (-10, 2.25)
  line L166 (-10, 17.25) -> (-20.5, 17.25)
  line L167 (-20.5, 17.25) -> (-20.5, 27.75)
  line L168 (-20.5, 27.75) -> (-10, 27.75)
  line L169 (-10, 27.75) -> (-10, 17.25)
  line L170 (-10, 32.25) -> (-20.5, 32.25)
  line L171 (-20.5, 32.25) -> (-20.5, 42.75)
  line L172 (-20.5, 42.75) -> (-10, 42.75)
  line L173 (-10, 42.75) -> (-10, 32.25)
  line L174 (-10, 47.25) -> (-20.5, 47.25)
  line L175 (-20.5, 47.25) -> (-20.5, 57.75)
  line L176 (-20.5, 57.75) -> (-10, 57.75)
  line L177 (-10, 57.75) -> (-10, 47.25)
  line L178 (-10, 62.25) -> (-20.5, 62.25)
  line L179 (-20.5, 62.25) -> (-20.5, 72.75)
  line L180 (-20.5, 72.75) -> (-10, 72.75)
  line L181 (-10, 72.75) -> (-10, 62.25)
  line L182 (-10, 77.25) -> (-20.5, 77.25)
  line L183 (-20.5, 77.25) -> (-20.5, 87.75)
  line L184 (-20.5, 87.75) -> (-10, 87.75)
  line L185 (-10, 87.75) -> (-10, 77.25)
  line L186 (-10, 92.25) -> (-20.5, 92.25)
  line L187 (-20.5, 92.25) -> (-20.5, 102.75)
  line L188 (-20.5, 102.75) -> (-10, 102.75)
  line L189 (-10, 102.75) -> (-10, 92.25)
  line L190 (-10, 107.25) -> (-20.5, 107.25)
  line L191 (-20.5, 107.25) -> (-20.5, 117.75)
  line L192 (-20.5, 117.75) -> (-10, 117.75)
  line L193 (-10, 117.75) -> (-10, 107.25)
  line L194 (5, -117.75) -> (-5.5, -117.75)
  line L195 (-5.5, -117.75) -> (-5.5, -107.25)
  line L196 (-5.5, -107.25) -> (5, -107.25)
  line L197 (5, -107.25) -> (5, -117.75)
  line L198 (5, -102.75) -> (-5.5, -102.75)
  line L199 (-5.5, -102.75) -> (-5.5, -92.25)
  line L200 (-5.5, -92.25) -> (5, -92.25)
  line L201 (5, -92.25) -> (5, -102.75)
  line L202 (5, -87.75) -> (-5.5, -87.75)
  line L203 (-5.5, -87.75) -> (-5.5, -77.25)
  line L204 (-5.5, -77.25) -> (5, -77.25)
  line L205 (5, -77.25) -> (5, -87.75)
  line L206 (5, -72.75) -> (-5.5, -72.75)
  line L207 (-5.5, -72.75) -> (-5.5, -62.25)
  line L208 (-5.5, -62.25) -> (5, -62.25)
  line L209 (5, -62.25) -> (5, -72.75)
  line L210 (5, -57.75) -> (-5.5, -57.75)
  line L211 (-5.5, -57.75) -> (-5.5, -47.25)
  line L212 (-5.5, -47.25) -> (5, -47.25)
  line L213 (5, -47.25) -> (5, -57.75)
  line L214 (5, -42.75) -> (-5.5, -42.75)
  line L215 (-5.5, -42.75) -> (-5.5, -32.25)
  line L216 (-5.5, -32.25) -> (5, -32.25)
  line L217 (5, -32.25) -> (5, -42.75)
  line L218 (5, -27.75) -> (-5.5, -27.75)
  line L219 (-5.5, -27.75) -> (-5.5, -17.25)
  line L220 (-5.5, -17.25) -> (5, -17.25)
  line L221 (5, -17.25) -> (5, -27.75)
  line L222 (5, -12.75) -> (-5.5, -12.75)
  line L223 (-5.5, -12.75) -> (-5.5, -2.25)
  line L224 (-5.5, -2.25) -> (5, -2.25)
  line L225 (5, -2.25) -> (5, -12.75)
  line L226 (5, 2.25) -> (-5.5, 2.25)
  line L227 (-5.5, 2.25) -> (-5.5, 12.75)
  line L228 (-5.5, 12.75) -> (5, 12.75)
  line L229 (5, 12.75) -> (5, 2.25)
  line L230 (5, 17.25) -> (-5.5, 17.25)
  line L231 (-5.5, 17.25) -> (-5.5, 27.75)
  line L232 (-5.5, 27.75) -> (5, 27.75)
  line L233 (5, 27.75) -> (5, 17.25)
  line L234 (5, 32.25) -> (-5.5, 32.25)
  line L235 (-5.5, 32.25) -> (-5.5, 42.75)
  line L236 (-5.5, 42.75) -> (5, 42.75)
  line L237 (5, 42.75) -> (5, 32.25)
  line L238 (5, 47.25) -> (-5.5, 47.25)
  line L239 (-5.5, 47.25) -> (-5.5, 57.75)
  line L240 (-5.5, 57.75) -> (5, 57.75)
  line L241 (5, 57.75) -> (5, 47.25)
  line L242 (5, 62.25) -> (-5.5, 62.25)
  line L243 (-5.5, 62.25) -> (-5.5, 72.75)
  line L244 (-5.5, 72.75) -> (5, 72.75)
  line L245 (5, 72.75) -> (5, 62.25)
  line L246 (5, 77.25) -> (-5.5, 77.25)
  line L247 (-5.5, 77.25) -> (-5.5, 87.75)
  line L248 (-5.5, 87.75) -> (5, 87.75)
  line L249 (5, 87.75) -> (5, 77.25)
  line L250 (5, 92.25) -> (-5.5, 92.25)
  line L251 (-5.5, 92.25) -> (-5.5, 102.75)
  line L252 (-5.5, 102.75) -> (5, 102.75)
  line L253 (5, 102.75) -> (5, 92.25)
  line L254 (5, 107.25) -> (-5.5, 107.25)
  line L255 (-5.5, 107.25) -> (-5.5, 117.75)
  line L256 (-5.5, 117.75) -> (5, 117.75)
  line L257 (5, 117.75) -> (5, 107.25)
  line L258 (20, -117.75) -> (9.5, -117.75)
  line L259 (9.5, -117.75) -> (9.5, -107.25)
  line L260 (9.5, -107.25) -> (20, -107.25)
  line L261 (20, -107.25) -> (20, -117.75)
  line L262 (20, -102.75) -> (9.5, -102.75)
  line L263 (9.5, -102.75) -> (9.5, -92.25)
  line L264 (9.5, -92.25) -> (20, -92.25)
  line L265 (20, -92.25) -> (20, -102.75)
  line L266 (20, -87.75) -> (9.5, -87.75)
  line L267 (9.5, -87.75) -> (9.5, -77.25)
  line L268 (9.5, -77.25) -> (20, -77.25)
  line L269 (20, -77.25) -> (20, -87.75)
  line L270 (20, -72.75) -> (9.5, -72.75)
  line L271 (9.5, -72.75) -> (9.5, -62.25)
  line L272 (9.5, -62.25) -> (20, -62.25)
  line L273 (20, -62.25) -> (20, -72.75)
  line L274 (20, -57.75) -> (9.5, -57.75)
  line L275 (9.5, -57.75) -> (9.5, -47.25)
  line L276 (9.5, -47.25) -> (20, -47.25)
  line L277 (20, -47.25) -> (20, -57.75)
  line L278 (20, -42.75) -> (9.5, -42.75)
  line L279 (9.5, -42.75) -> (9.5, -32.25)
  line L280 (9.5, -32.25) -> (20, -32.25)
  line L281 (20, -32.25) -> (20, -42.75)
  line L282 (20, -27.75) -> (9.5, -27.75)
  line L283 (9.5, -27.75) -> (9.5, -17.25)
  line L284 (9.5, -17.25) -> (20, -17.25)
  line L285 (20, -17.25) -> (20, -27.75)
  line L286 (20, -12.75) -> (9.5, -12.75)
  line L287 (9.5, -12.75) -> (9.5, -2.25)
  line L288 (9.5, -2.25) -> (20, -2.25)
  line L289 (20, -2.25) -> (20, -12.75)
  line L290 (20, 2.25) -> (9.5, 2.25)
  line L291 (9.5, 2.25) -> (9.5, 12.75)
  line L292 (9.5, 12.75) -> (20, 12.75)
  line L293 (20, 12.75) -> (20, 2.25)
  line L294 (20, 17.25) -> (9.5, 17.25)
  line L295 (9.5, 17.25) -> (9.5, 27.75)
  line L296 (9.5, 27.75) -> (20, 27.75)
  line L297 (20, 27.75) -> (20, 17.25)
  line L298 (20, 32.25) -> (9.5, 32.25)
  line L299 (9.5, 32.25) -> (9.5, 42.75)
  line L300 (9.5, 42.75) -> (20, 42.75)
  line L301 (20, 42.75) -> (20, 32.25)
  line L302 (20, 47.25) -> (9.5, 47.25)
  line L303 (9.5, 47.25) -> (9.5, 57.75)
  line L304 (9.5, 57.75) -> (20, 57.75)
  line L305 (20, 57.75) -> (20, 47.25)
  line L306 (20, 62.25) -> (9.5, 62.25)
  line L307 (9.5, 62.25) -> (9.5, 72.75)
  line L308 (9.5, 72.75) -> (20, 72.75)
  line L309 (20, 72.75) -> (20, 62.25)
  line L310 (20, 77.25) -> (9.5, 77.25)
  line L311 (9.5, 77.25) -> (9.5, 87.75)
  line L312 (9.5, 87.75) -> (20, 87.75)
  line L313 (20, 87.75) -> (20, 77.25)
  line L314 (20, 92.25) -> (9.5, 92.25)
  line L315 (9.5, 92.25) -> (9.5, 102.75)
  line L316 (9.5, 102.75) -> (20, 102.75)
  line L317 (20, 102.75) -> (20, 92.25)
  line L318 (20, 107.25) -> (9.5, 107.25)
  line L319 (9.5, 107.25) -> (9.5, 117.75)
  line L320 (9.5, 117.75) -> (20, 117.75)
  line L321 (20, 117.75) -> (20, 107.25)
  line L322 (35, -117.75) -> (24.5, -117.75)
  line L323 (24.5, -117.75) -> (24.5, -107.25)
  line L324 (24.5, -107.25) -> (35, -107.25)
  line L325 (35, -107.25) -> (35, -117.75)
  line L326 (35, -102.75) -> (24.5, -102.75)
  line L327 (24.5, -102.75) -> (24.5, -92.25)
  line L328 (24.5, -92.25) -> (35, -92.25)
  line L329 (35, -92.25) -> (35, -102.75)
  line L330 (35, -87.75) -> (24.5, -87.75)
  line L331 (24.5, -87.75) -> (24.5, -77.25)
  line L332 (24.5, -77.25) -> (35, -77.25)
  line L333 (35, -77.25) -> (35, -87.75)
  line L334 (35, -72.75) -> (24.5, -72.75)
  line L335 (24.5, -72.75) -> (24.5, -62.25)
  line L336 (24.5, -62.25) -> (35, -62.25)
  line L337 (35, -62.25) -> (35, -72.75)
  line L338 (35, -57.75) -> (24.5, -57.75)
  line L339 (24.5, -57.75) -> (24.5, -47.25)
  line L340 (24.5, -47.25) -> (35, -47.25)
  line L341 (35, -47.25) -> (35, -57.75)
  line L342 (35, -42.75) -> (24.5, -42.75)
  line L343 (24.5, -42.75) -> (24.5, -32.25)
  line L344 (24.5, -32.25) -> (35, -32.25)
  line L345 (35, -32.25) -> (35, -42.75)
  line L346 (35, -27.75) -> (24.5, -27.75)
  line L347 (24.5, -27.75) -> (24.5, -17.25)
  line L348 (24.5, -17.25) -> (35, -17.25)
  line L349 (35, -17.25) -> (35, -27.75)
  line L350 (35, -12.75) -> (24.5, -12.75)
  line L351 (24.5, -12.75) -> (24.5, -2.25)
  line L352 (24.5, -2.25) -> (35, -2.25)
  line L353 (35, -2.25) -> (35, -12.75)
  line L354 (35, 2.25) -> (24.5, 2.25)
  line L355 (24.5, 2.25) -> (24.5, 12.75)
  line L356 (24.5, 12.75) -> (35, 12.75)
  line L357 (35, 12.75) -> (35, 2.25)
  line L358 (35, 17.25) -> (24.5, 17.25)
  line L359 (24.5, 17.25) -> (24.5, 27.75)
  line L360 (24.5, 27.75) -> (35, 27.75)
  line L361 (35, 27.75) -> (35, 17.25)
  line L362 (35, 32.25) -> (24.5, 32.25)
  line L363 (24.5, 32.25) -> (24.5, 42.75)
  line L364 (24.5, 42.75) -> (35, 42.75)
  line L365 (35, 42.75) -> (35, 32.25)
  line L366 (35, 47.25) -> (24.5, 47.25)
  line L367 (24.5, 47.25) -> (24.5, 57.75)
  line L368 (24.5, 57.75) -> (35, 57.75)
  line L369 (35, 57.75) -> (35, 47.25)
  line L370 (35, 62.25) -> (24.5, 62.25)
  line L371 (24.5, 62.25) -> (24.5, 72.75)
  line L372 (24.5, 72.75) -> (35, 72.75)
  line L373 (35, 72.75) -> (35, 62.25)
  line L374 (35, 77.25) -> (24.5, 77.25)
  line L375 (24.5, 77.25) -> (24.5, 87.75)
  line L376 (24.5, 87.75) -> (35, 87.75)
  line L377 (35, 87.75) -> (35, 77.25)
  line L378 (35, 92.25) -> (24.5, 92.25)
  line L379 (24.5, 92.25) -> (24.5, 102.75)
  line L380 (24.5, 102.75) -> (35, 102.75)
  line L381 (35, 102.75) -> (35, 92.25)
  line L382 (35, 107.25) -> (24.5, 107.25)
  line L383 (24.5, 107.25) -> (24.5, 117.75)
  line L384 (24.5, 117.75) -> (35, 117.75)
  line L385 (35, 117.75) -> (35, 107.25)
  line L386 (50, -117.75) -> (39.5, -117.75)
  line L387 (39.5, -117.75) -> (39.5, -107.25)
  line L388 (39.5, -107.25) -> (50, -107.25)
  line L389 (50, -107.25) -> (50, -117.75)
  line L390 (50, -102.75) -> (39.5, -102.75)
  line L391 (39.5, -102.75) -> (39.5, -92.25)
  line L392 (39.5, -92.25) -> (50, -92.25)
  line L393 (50, -92.25) -> (50, -102.75)
  line L394 (50, -87.75) -> (39.5, -87.75)
  line L395 (39.5, -87.75) -> (39.5, -77.25)
  line L396 (39.5, -77.25) -> (50, -77.25)
  line L397 (50, -77.25) -> (50, -87.75)
  line L398 (50, -72.75) -> (39.5, -72.75)
  line L399 (39.5, -72.75) -> (39.5, -62.25)
  line L400 (39.5, -62.25) -> (50, -62.25)
  line L401 (50, -62.25) -> (50, -72.75)
  line L402 (50, -57.75) -> (39.5, -57.75)
  line L403 (39.5, -57.75) -> (39.5, -47.25)
  line L404 (39.5, -47.25) -> (50, -47.25)
  line L405 (50, -47.25) -> (50, -57.75)
  line L406 (50, -42.75) -> (39.5, -42.75)
  line L407 (39.5, -42.75) -> (39.5, -32.25)
  line L408 (39.5, -32.25) -> (50, -32.25)
  line L409 (50, -32.25) -> (50, -42.75)
  line L410 (50, -27.75) -> (39.5, -27.75)
  line L411 (39.5, -27.75) -> (39.5, -17.25)
  line L412 (39.5, -17.25) -> (50, -17.25)
  line L413 (50, -17.25) -> (50, -27.75)
  line L414 (50, -12.75) -> (39.5, -12.75)
  line L415 (39.5, -12.75) -> (39.5, -2.25)
  line L416 (39.5, -2.25) -> (50, -2.25)
  line L417 (50, -2.25) -> (50, -12.75)
  line L418 (50, 2.25) -> (39.5, 2.25)
  line L419 (39.5, 2.25) -> (39.5, 12.75)
  line L420 (39.5, 12.75) -> (50, 12.75)
  line L421 (50, 12.75) -> (50, 2.25)
  line L422 (50, 17.25) -> (39.5, 17.25)
  line L423 (39.5, 17.25) -> (39.5, 27.75)
  line L424 (39.5, 27.75) -> (50, 27.75)
  line L425 (50, 27.75) -> (50, 17.25)
  line L426 (50, 32.25) -> (39.5, 32.25)
  line L427 (39.5, 32.25) -> (39.5, 42.75)
  line L428 (39.5, 42.75) -> (50, 42.75)
  line L429 (50, 42.75) -> (50, 32.25)
  line L430 (50, 47.25) -> (39.5, 47.25)
  line L431 (39.5, 47.25) -> (39.5, 57.75)
  line L432 (39.5, 57.75) -> (50, 57.75)
  line L433 (50, 57.75) -> (50, 47.25)
  line L434 (50, 62.25) -> (39.5, 62.25)
  line L435 (39.5, 62.25) -> (39.5, 72.75)
  line L436 (39.5, 72.75) -> (50, 72.75)
  line L437 (50, 72.75) -> (50, 62.25)
  line L438 (50, 77.25) -> (39.5, 77.25)
  line L439 (39.5, 77.25) -> (39.5, 87.75)
  line L440 (39.5, 87.75) -> (50, 87.75)
  line L441 (50, 87.75) -> (50, 77.25)
  line L442 (50, 92.25) -> (39.5, 92.25)
  line L443 (39.5, 92.25) -> (39.5, 102.75)
  line L444 (39.5, 102.75) -> (50, 102.75)
  line L445 (50, 102.75) -> (50, 92.25)
  line L446 (50, 107.25) -> (39.5, 107.25)
  line L447 (39.5, 107.25) -> (39.5, 117.75)
  line L448 (39.5, 117.75) -> (50, 117.75)
  line L449 (50, 117.75) -> (50, 107.25)
  line L450 (24.5, -87.75) -> (50, -87.75)
  line L451 (50, -87.75) -> (50, -77.25)
  line L452 (50, -77.25) -> (24.5, -77.25)
  line L453 (24.5, -77.25) -> (24.5, -87.75)
  line L454 (24.5, -72.75) -> (50, -72.75)
  line L455 (50, -72.75) -> (50, -62.25)
  line L456 (50, -62.25) -> (24.5, -62.25)
  line L457 (24.5, -62.25) -> (24.5, -72.75)
  line L458 (24.5, -57.75) -> (50, -57.75)
  line L459 (50, -57.75) -> (50, -47.25)
  line L460 (50, -47.25) -> (24.5, -47.25)
  line L461 (24.5, -47.25) -> (24.5, -57.75)
  line L462 (24.5, -42.75) -> (50, -42.75)
  line L463 (50, -42.75) -> (50, -32.25)
  line L464 (50, -32.25) -> (24.5, -32.25)
  line L465 (24.5, -32.25) -> (24.5, -42.75)
  line L466 (24.5, -27.75) -> (50, -27.75)
  line L467 (50, -27.75) -> (50, -17.25)
  line L468 (50, -17.25) -> (24.5, -17.25)
  line L469 (24.5, -17.25) -> (24.5, -27.75)
  line L470 (24.5, -12.75) -> (50, -12.75)
  line L471 (50, -12.75) -> (50, -2.25)
  line L472 (50, -2.25) -> (24.5, -2.25)
  line L473 (24.5, -2.25) -> (24.5, -12.75)
  line L474 (24.5, 2.25) -> (50, 2.25)
  line L475 (50, 2.25) -> (50, 12.75)
  line L476 (50, 12.75) -> (24.5, 12.75)
  line L477 (24.5, 12.75) -> (24.5, 2.25)
  line L478 (24.5, 17.25) -> (50, 17.25)
  line L479 (50, 17.25) -> (50, 27.75)
  line L480 (50, 27.75) -> (24.5, 27.75)
  line L481 (24.5, 27.75) -> (24.5, 17.25)
  line L482 (24.5, 32.25) -> (50, 32.25)
  line L483 (50, 32.25) -> (50, 42.75)
  line L484 (50, 42.75) -> (24.5, 42.75)
  line L485 (24.5, 42.75) -> (24.5, 32.25)
  line L486 (24.5, 47.25) -> (50, 47.25)
  line L487 (50, 47.25) -> (50, 57.75)
  line L488 (50, 57.75) -> (24.5, 57.75)
  line L489 (24.5, 57.75) -> (24.5, 47.25)
  line L490 (24.5, 62.25) -> (50, 62.25)
  line L491 (50, 62.25) -> (50, 72.75)
  line L492 (50, 72.75) -> (24.5, 72.75)
  line L493 (24.5, 72.75) -> (24.5, 62.25)
  line L494 (24.5, 77.25) -> (50, 77.25)
  line L495 (50, 77.25) -> (50, 87.75)
  line L496 (50, 87.75) -> (24.5, 87.75)
  line L497 (24.5, 87.75) -> (24.5, 77.25)
  line L498 (24.5, 92.25) -> (50, 92.25)
  line L499 (50, 92.25) -> (50, 102.75)
  line L500 (50, 102.75) -> (24.5, 102.75)
  line L501 (24.5, 102.75) -> (24.5, 92.25)
  line L502 (24.5, 107.25) -> (50, 107.25)
  line L503 (50, 107.25) -> (50, 117.75)
  line L504 (50, 117.75) -> (24.5, 117.75)
  line L505 (24.5, 117.75) -> (24.5, 107.25)
  line L506 (9.5, -87.75) -> (20, -87.75)
  line L507 (20, -87.75) -> (20, -69.75)
  line L508 (20, -69.75) -> (9.5, -69.75)
  line L509 (9.5, -69.75) -> (9.5, -87.75)
  line L510 (9.5, -47.25) -> (20, -47.25)
  line L511 (20, -47.25) -> (20, -65.25)
  line L512 (20, -65.25) -> (9.5, -65.25)
  line L513 (9.5, -65.25) -> (9.5, -47.25)
  line L514 (9.5, -42.75) -> (20, -42.75)
  line L515 (20, -42.75) -> (20, -24.75)
  line L516 (20, -24.75) -> (9.5, -24.75)
  line L517 (9.5, -24.75) -> (9.5, -42.75)
  line L518 (9.5, -20.25) -> (20, -20.25)
  line L519 (20, -20.25) -> (20, -9.75)
  line L520 (20, -9.75) -> (9.5, -9.75)
  line L521 (9.5, -9.75) -> (9.5, -20.25)